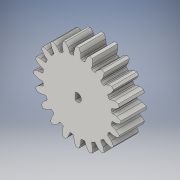
# Autodesk Inventor part: Pinion Gear
Saved by Autodesk Inventor 2016 (Build 200138000, 138)
## iProperties
Created: 2016-04-02
Part Number: Pinion Gear
Material: Generic
Document SubType Name: Modeling
Designer: amycroft3
Density: 1 g/cm^3
Appearance: White
Author: amycroft3
Autodesk Inventor part; units mm, degrees
ref_plane "YZ Plane" through (0, 0, 0) normal (1, 0, 0) x (0, 1, 0)
ref_plane "XZ Plane" through (0, 0, 0) normal (0, 1, 0) x (-1, 0, 0)
ref_plane "XY Plane" through (0, 0, 0) normal (0, 0, 1) x (1, 0, 0)
sketch "Sketch2" plane through (0, 0, 0) normal (0, 0, 1) x (1, 0, 0)
  spline S0 degree 3 poles (-17.8641, 1.7548) (-18.4191, 1.7613) (-18.9748, 1.7752) (-19.5187, 1.6705) (-19.6593, 1.6434) (-19.799, 1.6083) (-19.9383, 1.5692) knots 0 0 0 0 0.001655 0.001655 0.001655 0.002082 0.002082 0.002082 0.002082
  arc A0 (-19.9383, 1.5692) -> (-19.9383, -1.5692) centre (0, 0) ccw
  spline S1 degree 3 poles (-19.9383, -1.5692) (-19.7998, -1.6081) (-19.6596, -1.6433) (-19.5187, -1.6705) (-18.9722, -1.7757) (-18.418, -1.7613) (-17.8641, -1.7548) knots 0.002234 0.002234 0.002234 0.002234 0.002666 0.002666 0.002666 0.004341 0.004341 0.004341 0.004341
  arc A1 (-17.3622, -2.1921) -> (-17.8641, -1.7548) centre (-17.8582, -2.2548) ccw
  arc A2 (-17.3622, -2.1921) -> (-17.1898, -3.2804) centre (0, 0) ccw
  arc A3 (-17.532, -3.8514) -> (-17.1898, -3.2804) centre (-17.6809, -3.3741) ccw
  spline S2 degree 3 poles (-17.532, -3.8514) (-18.0619, -4.0167) (-18.5947, -4.1752) (-19.0796, -4.4429) (-19.2049, -4.5121) (-19.327, -4.5887) (-19.4474, -4.6689) knots 0 0 0 0 0.001655 0.001655 0.001655 0.002082 0.002082 0.002082 0.002082
  arc A4 (-19.4474, -4.6689) -> (-18.4776, -7.6537) centre (0, 0) ccw
  spline S3 degree 3 poles (-18.4776, -7.6537) (-18.3338, -7.6478) (-18.1895, -7.6381) (-18.0472, -7.6203) (-17.4949, -7.5515) (-16.9723, -7.3666) (-16.4475, -7.1892) knots 0.002234 0.002234 0.002234 0.002234 0.002666 0.002666 0.002666 0.004341 0.004341 0.004341 0.004341
  arc A5 (-15.835, -7.45) -> (-16.4475, -7.1892) centre (-16.2874, -7.6629) ccw
  arc A6 (-15.835, -7.45) -> (-15.3348, -8.4317) centre (0, 0) ccw
  arc A7 (-15.4838, -9.0806) -> (-15.3348, -8.4317) centre (-15.7729, -8.6727) ccw
  spline S4 degree 3 poles (-15.4838, -9.0806) (-15.9366, -9.4015) (-16.3944, -9.7169) (-16.7729, -10.1214) (-16.8707, -10.2259) (-16.9631, -10.3364) (-17.0528, -10.45) knots 0 0 0 0 0.001655 0.001655 0.001655 0.002082 0.002082 0.002082 0.002082
  arc A8 (-17.0528, -10.45) -> (-15.2081, -12.989) centre (0, 0) ccw
  spline S5 degree 3 poles (-15.2081, -12.989) (-15.0732, -12.939) (-14.939, -12.8851) (-14.8091, -12.8243) (-14.3051, -12.5882) (-13.8652, -12.2508) (-13.4209, -11.9199) knots 0.002234 0.002234 0.002234 0.002234 0.002666 0.002666 0.002666 0.004341 0.004341 0.004341 0.004341
  arc A9 (-12.7578, -11.9787) -> (-13.4209, -11.9199) centre (-13.1223, -12.3209) ccw
  arc A10 (-12.7578, -11.9787) -> (-11.9787, -12.7578) centre (0, 0) ccw
  arc A11 (-11.9199, -13.4209) -> (-11.9787, -12.7578) centre (-12.3209, -13.1223) ccw
  spline S6 degree 3 poles (-11.9199, -13.4209) (-12.2514, -13.8661) (-12.5893, -14.3075) (-12.8243, -14.8091) (-12.885, -14.9387) (-12.9387, -15.0724) (-12.989, -15.2081) knots 0 0 0 0 0.001655 0.001655 0.001655 0.002082 0.002082 0.002082 0.002082
  arc A12 (-12.989, -15.2081) -> (-10.45, -17.0528) centre (0, 0) ccw
  spline S7 degree 3 poles (-10.45, -17.0528) (-10.3371, -16.9636) (-10.2261, -16.8708) (-10.1214, -16.7729) (-9.715, -16.3926) (-9.4009, -15.9357) (-9.0806, -15.4838) knots 0.002234 0.002234 0.002234 0.002234 0.002666 0.002666 0.002666 0.004341 0.004341 0.004341 0.004341
  arc A13 (-8.4317, -15.3348) -> (-9.0806, -15.4838) centre (-8.6727, -15.7729) ccw
  arc A14 (-8.4317, -15.3348) -> (-7.45, -15.835) centre (0, 0) ccw
  arc A15 (-7.1892, -16.4475) -> (-7.45, -15.835) centre (-7.6629, -16.2874) ccw
  spline S8 degree 3 poles (-7.1892, -16.4475) (-7.3669, -16.9733) (-7.5519, -17.4975) (-7.6203, -18.0472) (-7.638, -18.1892) (-7.6478, -18.333) (-7.6537, -18.4776) knots 0 0 0 0 0.001655 0.001655 0.001655 0.002082 0.002082 0.002082 0.002082
  arc A16 (-7.6537, -18.4776) -> (-4.6689, -19.4474) centre (0, 0) ccw
  spline S9 degree 3 poles (-4.6689, -19.4474) (-4.5891, -19.3276) (-4.5122, -19.2052) (-4.4429, -19.0796) (-4.1739, -18.5923) (-4.0164, -18.0608) (-3.8514, -17.532) knots 0.002234 0.002234 0.002234 0.002234 0.002666 0.002666 0.002666 0.004341 0.004341 0.004341 0.004341
  arc A17 (-3.2804, -17.1898) -> (-3.8514, -17.532) centre (-3.3741, -17.6809) ccw
  arc A18 (-3.2804, -17.1898) -> (-2.1921, -17.3622) centre (0, 0) ccw
  arc A19 (-1.7548, -17.8641) -> (-2.1921, -17.3622) centre (-2.2548, -17.8582) ccw
  spline S10 degree 3 poles (-1.7548, -17.8641) (-1.7613, -18.4191) (-1.7752, -18.9748) (-1.6705, -19.5187) (-1.6434, -19.6593) (-1.6083, -19.799) (-1.5692, -19.9383) knots 0 0 0 0 0.001655 0.001655 0.001655 0.002082 0.002082 0.002082 0.002082
  arc A20 (-1.5692, -19.9383) -> (1.5692, -19.9383) centre (0, 0) ccw
  spline S11 degree 3 poles (1.5692, -19.9383) (1.6081, -19.7998) (1.6433, -19.6596) (1.6705, -19.5187) (1.7757, -18.9722) (1.7613, -18.418) (1.7548, -17.8641) knots 0.002234 0.002234 0.002234 0.002234 0.002666 0.002666 0.002666 0.004341 0.004341 0.004341 0.004341
  arc A21 (2.1921, -17.3622) -> (1.7548, -17.8641) centre (2.2548, -17.8582) ccw
  arc A22 (2.1921, -17.3622) -> (3.2804, -17.1898) centre (0, 0) ccw
  arc A23 (3.8514, -17.532) -> (3.2804, -17.1898) centre (3.3741, -17.6809) ccw
  spline S12 degree 3 poles (3.8514, -17.532) (4.0167, -18.0619) (4.1752, -18.5947) (4.4429, -19.0796) (4.5121, -19.2049) (4.5887, -19.327) (4.6689, -19.4474) knots 0 0 0 0 0.001655 0.001655 0.001655 0.002082 0.002082 0.002082 0.002082
  arc A24 (4.6689, -19.4474) -> (7.6537, -18.4776) centre (0, 0) ccw
  spline S13 degree 3 poles (7.6537, -18.4776) (7.6478, -18.3338) (7.6381, -18.1895) (7.6203, -18.0472) (7.5515, -17.4949) (7.3666, -16.9723) (7.1892, -16.4475) knots 0.002234 0.002234 0.002234 0.002234 0.002666 0.002666 0.002666 0.004341 0.004341 0.004341 0.004341
  arc A25 (7.45, -15.835) -> (7.1892, -16.4475) centre (7.6629, -16.2874) ccw
  arc A26 (7.45, -15.835) -> (8.4317, -15.3348) centre (0, 0) ccw
  arc A27 (9.0806, -15.4838) -> (8.4317, -15.3348) centre (8.6727, -15.7729) ccw
  spline S14 degree 3 poles (9.0806, -15.4838) (9.4015, -15.9366) (9.7169, -16.3944) (10.1214, -16.7729) (10.2259, -16.8707) (10.3364, -16.9631) (10.45, -17.0528) knots 0 0 0 0 0.001655 0.001655 0.001655 0.002082 0.002082 0.002082 0.002082
  arc A28 (10.45, -17.0528) -> (12.989, -15.2081) centre (0, 0) ccw
  spline S15 degree 3 poles (12.989, -15.2081) (12.939, -15.0732) (12.8851, -14.939) (12.8243, -14.8091) (12.5882, -14.3051) (12.2508, -13.8652) (11.9199, -13.4209) knots 0.002234 0.002234 0.002234 0.002234 0.002666 0.002666 0.002666 0.004341 0.004341 0.004341 0.004341
  arc A29 (11.9787, -12.7578) -> (11.9199, -13.4209) centre (12.3209, -13.1223) ccw
  arc A30 (11.9787, -12.7578) -> (12.7578, -11.9787) centre (0, 0) ccw
  arc A31 (13.4209, -11.9199) -> (12.7578, -11.9787) centre (13.1223, -12.3209) ccw
  spline S16 degree 3 poles (13.4209, -11.9199) (13.8661, -12.2514) (14.3075, -12.5893) (14.8091, -12.8243) (14.9387, -12.885) (15.0724, -12.9387) (15.2081, -12.989) knots 0 0 0 0 0.001655 0.001655 0.001655 0.002082 0.002082 0.002082 0.002082
  arc A32 (15.2081, -12.989) -> (17.0528, -10.45) centre (0, 0) ccw
  spline S17 degree 3 poles (17.0528, -10.45) (16.9636, -10.3371) (16.8708, -10.2261) (16.7729, -10.1214) (16.3926, -9.715) (15.9357, -9.4009) (15.4838, -9.0806) knots 0.002234 0.002234 0.002234 0.002234 0.002666 0.002666 0.002666 0.004341 0.004341 0.004341 0.004341
  arc A33 (15.3348, -8.4317) -> (15.4838, -9.0806) centre (15.7729, -8.6727) ccw
  arc A34 (15.3348, -8.4317) -> (15.835, -7.45) centre (0, 0) ccw
  arc A35 (16.4475, -7.1892) -> (15.835, -7.45) centre (16.2874, -7.6629) ccw
  spline S18 degree 3 poles (16.4475, -7.1892) (16.9733, -7.3669) (17.4975, -7.5519) (18.0472, -7.6203) (18.1892, -7.638) (18.333, -7.6478) (18.4776, -7.6537) knots 0 0 0 0 0.001655 0.001655 0.001655 0.002082 0.002082 0.002082 0.002082
  arc A36 (18.4776, -7.6537) -> (19.4474, -4.6689) centre (0, 0) ccw
  spline S19 degree 3 poles (19.4474, -4.6689) (19.3276, -4.5891) (19.2052, -4.5122) (19.0796, -4.4429) (18.5923, -4.1739) (18.0608, -4.0164) (17.532, -3.8514) knots 0.002234 0.002234 0.002234 0.002234 0.002666 0.002666 0.002666 0.004341 0.004341 0.004341 0.004341
  arc A37 (17.1898, -3.2804) -> (17.532, -3.8514) centre (17.6809, -3.3741) ccw
  arc A38 (17.1898, -3.2804) -> (17.3622, -2.1921) centre (0, 0) ccw
  arc A39 (17.8641, -1.7548) -> (17.3622, -2.1921) centre (17.8582, -2.2548) ccw
  spline S20 degree 3 poles (17.8641, -1.7548) (18.4191, -1.7613) (18.9748, -1.7752) (19.5187, -1.6705) (19.6593, -1.6434) (19.799, -1.6083) (19.9383, -1.5692) knots 0 0 0 0 0.001655 0.001655 0.001655 0.002082 0.002082 0.002082 0.002082
  arc A40 (19.9383, -1.5692) -> (19.9383, 1.5692) centre (0, 0) ccw
  spline S21 degree 3 poles (19.9383, 1.5692) (19.7998, 1.6081) (19.6596, 1.6433) (19.5187, 1.6705) (18.9722, 1.7757) (18.418, 1.7613) (17.8641, 1.7548) knots 0.002234 0.002234 0.002234 0.002234 0.002666 0.002666 0.002666 0.004341 0.004341 0.004341 0.004341
  arc A41 (17.3622, 2.1921) -> (17.8641, 1.7548) centre (17.8582, 2.2548) ccw
  arc A42 (17.3622, 2.1921) -> (17.1898, 3.2804) centre (0, 0) ccw
  arc A43 (17.532, 3.8514) -> (17.1898, 3.2804) centre (17.6809, 3.3741) ccw
  spline S22 degree 3 poles (17.532, 3.8514) (18.0619, 4.0167) (18.5947, 4.1752) (19.0796, 4.4429) (19.2049, 4.5121) (19.327, 4.5887) (19.4474, 4.6689) knots 0 0 0 0 0.001655 0.001655 0.001655 0.002082 0.002082 0.002082 0.002082
  arc A44 (19.4474, 4.6689) -> (18.4776, 7.6537) centre (0, 0) ccw
  spline S23 degree 3 poles (18.4776, 7.6537) (18.3338, 7.6478) (18.1895, 7.6381) (18.0472, 7.6203) (17.4949, 7.5515) (16.9723, 7.3666) (16.4475, 7.1892) knots 0.002234 0.002234 0.002234 0.002234 0.002666 0.002666 0.002666 0.004341 0.004341 0.004341 0.004341
  arc A45 (15.835, 7.45) -> (16.4475, 7.1892) centre (16.2874, 7.6629) ccw
  arc A46 (15.835, 7.45) -> (15.3348, 8.4317) centre (0, 0) ccw
  arc A47 (15.4838, 9.0806) -> (15.3348, 8.4317) centre (15.7729, 8.6727) ccw
  spline S24 degree 3 poles (15.4838, 9.0806) (15.9366, 9.4015) (16.3944, 9.7169) (16.7729, 10.1214) (16.8707, 10.2259) (16.9631, 10.3364) (17.0528, 10.45) knots 0 0 0 0 0.001655 0.001655 0.001655 0.002082 0.002082 0.002082 0.002082
  arc A48 (17.0528, 10.45) -> (15.2081, 12.989) centre (0, 0) ccw
  spline S25 degree 3 poles (15.2081, 12.989) (15.0732, 12.939) (14.939, 12.8851) (14.8091, 12.8243) (14.3051, 12.5882) (13.8652, 12.2508) (13.4209, 11.9199) knots 0.002234 0.002234 0.002234 0.002234 0.002666 0.002666 0.002666 0.004341 0.004341 0.004341 0.004341
  arc A49 (12.7578, 11.9787) -> (13.4209, 11.9199) centre (13.1223, 12.3209) ccw
  arc A50 (12.7578, 11.9787) -> (11.9787, 12.7578) centre (0, 0) ccw
  arc A51 (11.9199, 13.4209) -> (11.9787, 12.7578) centre (12.3209, 13.1223) ccw
  spline S26 degree 3 poles (11.9199, 13.4209) (12.2514, 13.8661) (12.5893, 14.3075) (12.8243, 14.8091) (12.885, 14.9387) (12.9387, 15.0724) (12.989, 15.2081) knots 0 0 0 0 0.001655 0.001655 0.001655 0.002082 0.002082 0.002082 0.002082
  arc A52 (12.989, 15.2081) -> (10.45, 17.0528) centre (0, 0) ccw
  spline S27 degree 3 poles (10.45, 17.0528) (10.3371, 16.9636) (10.2261, 16.8708) (10.1214, 16.7729) (9.715, 16.3926) (9.4009, 15.9357) (9.0806, 15.4838) knots 0.002234 0.002234 0.002234 0.002234 0.002666 0.002666 0.002666 0.004341 0.004341 0.004341 0.004341
  arc A53 (8.4317, 15.3348) -> (9.0806, 15.4838) centre (8.6727, 15.7729) ccw
  arc A54 (8.4317, 15.3348) -> (7.45, 15.835) centre (0, 0) ccw
  arc A55 (7.1892, 16.4475) -> (7.45, 15.835) centre (7.6629, 16.2874) ccw
  spline S28 degree 3 poles (7.1892, 16.4475) (7.3669, 16.9733) (7.5519, 17.4975) (7.6203, 18.0472) (7.638, 18.1892) (7.6478, 18.333) (7.6537, 18.4776) knots 0 0 0 0 0.001655 0.001655 0.001655 0.002082 0.002082 0.002082 0.002082
  arc A56 (7.6537, 18.4776) -> (4.6689, 19.4474) centre (0, 0) ccw
  spline S29 degree 3 poles (4.6689, 19.4474) (4.5891, 19.3276) (4.5122, 19.2052) (4.4429, 19.0796) (4.1739, 18.5923) (4.0164, 18.0608) (3.8514, 17.532) knots 0.002234 0.002234 0.002234 0.002234 0.002666 0.002666 0.002666 0.004341 0.004341 0.004341 0.004341
  arc A57 (3.2804, 17.1898) -> (3.8514, 17.532) centre (3.3741, 17.6809) ccw
  arc A58 (3.2804, 17.1898) -> (2.1921, 17.3622) centre (0, 0) ccw
  arc A59 (1.7548, 17.8641) -> (2.1921, 17.3622) centre (2.2548, 17.8582) ccw
  spline S30 degree 3 poles (1.7548, 17.8641) (1.7613, 18.4191) (1.7752, 18.9748) (1.6705, 19.5187) (1.6434, 19.6593) (1.6083, 19.799) (1.5692, 19.9383) knots 0 0 0 0 0.001655 0.001655 0.001655 0.002082 0.002082 0.002082 0.002082
  arc A60 (1.5692, 19.9383) -> (-1.5692, 19.9383) centre (0, 0) ccw
  spline S31 degree 3 poles (-1.5692, 19.9383) (-1.6081, 19.7998) (-1.6433, 19.6596) (-1.6705, 19.5187) (-1.7757, 18.9722) (-1.7613, 18.418) (-1.7548, 17.8641) knots 0.002234 0.002234 0.002234 0.002234 0.002666 0.002666 0.002666 0.004341 0.004341 0.004341 0.004341
  arc A61 (-2.1921, 17.3622) -> (-1.7548, 17.8641) centre (-2.2548, 17.8582) ccw
  arc A62 (-2.1921, 17.3622) -> (-3.2804, 17.1898) centre (0, 0) ccw
  arc A63 (-3.8514, 17.532) -> (-3.2804, 17.1898) centre (-3.3741, 17.6809) ccw
  spline S32 degree 3 poles (-3.8514, 17.532) (-4.0167, 18.0619) (-4.1752, 18.5947) (-4.4429, 19.0796) (-4.5121, 19.2049) (-4.5887, 19.327) (-4.6689, 19.4474) knots 0 0 0 0 0.001655 0.001655 0.001655 0.002082 0.002082 0.002082 0.002082
  arc A64 (-4.6689, 19.4474) -> (-7.6537, 18.4776) centre (0, 0) ccw
  spline S33 degree 3 poles (-7.6537, 18.4776) (-7.6478, 18.3338) (-7.6381, 18.1895) (-7.6203, 18.0472) (-7.5515, 17.4949) (-7.3666, 16.9723) (-7.1892, 16.4475) knots 0.002234 0.002234 0.002234 0.002234 0.002666 0.002666 0.002666 0.004341 0.004341 0.004341 0.004341
  arc A65 (-7.45, 15.835) -> (-7.1892, 16.4475) centre (-7.6629, 16.2874) ccw
  arc A66 (-7.45, 15.835) -> (-8.4317, 15.3348) centre (0, 0) ccw
  arc A67 (-9.0806, 15.4838) -> (-8.4317, 15.3348) centre (-8.6727, 15.7729) ccw
  spline S34 degree 3 poles (-9.0806, 15.4838) (-9.4015, 15.9366) (-9.7169, 16.3944) (-10.1214, 16.7729) (-10.2259, 16.8707) (-10.3364, 16.9631) (-10.45, 17.0528) knots 0 0 0 0 0.001655 0.001655 0.001655 0.002082 0.002082 0.002082 0.002082
  arc A68 (-10.45, 17.0528) -> (-12.989, 15.2081) centre (0, 0) ccw
  spline S35 degree 3 poles (-12.989, 15.2081) (-12.939, 15.0732) (-12.8851, 14.939) (-12.8243, 14.8091) (-12.5882, 14.3051) (-12.2508, 13.8652) (-11.9199, 13.4209) knots 0.002234 0.002234 0.002234 0.002234 0.002666 0.002666 0.002666 0.004341 0.004341 0.004341 0.004341
  arc A69 (-11.9787, 12.7578) -> (-11.9199, 13.4209) centre (-12.3209, 13.1223) ccw
  arc A70 (-11.9787, 12.7578) -> (-12.7578, 11.9787) centre (0, 0) ccw
  arc A71 (-13.4209, 11.9199) -> (-12.7578, 11.9787) centre (-13.1223, 12.3209) ccw
  spline S36 degree 3 poles (-13.4209, 11.9199) (-13.8661, 12.2514) (-14.3075, 12.5893) (-14.8091, 12.8243) (-14.9387, 12.885) (-15.0724, 12.9387) (-15.2081, 12.989) knots 0 0 0 0 0.001655 0.001655 0.001655 0.002082 0.002082 0.002082 0.002082
  arc A72 (-15.2081, 12.989) -> (-17.0528, 10.45) centre (0, 0) ccw
  spline S37 degree 3 poles (-17.0528, 10.45) (-16.9636, 10.3371) (-16.8708, 10.2261) (-16.7729, 10.1214) (-16.3926, 9.715) (-15.9357, 9.4009) (-15.4838, 9.0806) knots 0.002234 0.002234 0.002234 0.002234 0.002666 0.002666 0.002666 0.004341 0.004341 0.004341 0.004341
  arc A73 (-15.3348, 8.4317) -> (-15.4838, 9.0806) centre (-15.7729, 8.6727) ccw
  arc A74 (-15.3348, 8.4317) -> (-15.835, 7.45) centre (0, 0) ccw
  arc A75 (-16.4475, 7.1892) -> (-15.835, 7.45) centre (-16.2874, 7.6629) ccw
  spline S38 degree 3 poles (-16.4475, 7.1892) (-16.9733, 7.3669) (-17.4975, 7.5519) (-18.0472, 7.6203) (-18.1892, 7.638) (-18.333, 7.6478) (-18.4776, 7.6537) knots 0 0 0 0 0.001655 0.001655 0.001655 0.002082 0.002082 0.002082 0.002082
  arc A76 (-18.4776, 7.6537) -> (-19.4474, 4.6689) centre (0, 0) ccw
  spline S39 degree 3 poles (-19.4474, 4.6689) (-19.3276, 4.5891) (-19.2052, 4.5122) (-19.0796, 4.4429) (-18.5923, 4.1739) (-18.0608, 4.0164) (-17.532, 3.8514) knots 0.002234 0.002234 0.002234 0.002234 0.002666 0.002666 0.002666 0.004341 0.004341 0.004341 0.004341
  arc A77 (-17.1898, 3.2804) -> (-17.532, 3.8514) centre (-17.6809, 3.3741) ccw
  arc A78 (-17.1898, 3.2804) -> (-17.3622, 2.1921) centre (0, 0) ccw
  arc A79 (-17.8641, 1.7548) -> (-17.3622, 2.1921) centre (-17.8582, 2.2548) ccw
  arc A80 (-15.2081, 12.989) -> (-17.0528, 10.45) centre (0, 0) ccw
  spline S40 degree 3 poles (-17.3812, 13.4869) (-17.0145, 13.4452) (-16.6476, 13.3855) (-15.9177, 13.2226) (-15.5627, 13.1203) (-15.2081, 12.989) knots -0.225972 -0.225972 -0.225972 -0.225972 -0.113443 -0.113443 -0.000001 -0.000001 -0.000001 -0.000001
  arc A81 (-17.3812, 13.4869) -> (-18.1978, 12.3628) centre (0, 0) ccw
  spline S41 degree 3 poles (-17.0528, 10.45) (-17.2873, 10.7466) (-17.4943, 11.0526) (-17.8748, 11.6964) (-18.045, 12.027) (-18.1978, 12.3628) knots -0.22563 -0.22563 -0.22563 -0.22563 -0.112359 -0.112359 0 0 0 0
  arc A82 (-18.4776, 7.6537) -> (-19.4474, 4.6689) centre (0, 0) ccw
  spline S42 degree 3 poles (-20.6981, 7.4557) (-20.3366, 7.5294) (-19.9691, 7.586) (-19.2247, 7.6566) (-18.8554, 7.669) (-18.4776, 7.6537) knots -0.225972 -0.225972 -0.225972 -0.225972 -0.113443 -0.113443 -0.000001 -0.000001 -0.000001 -0.000001
  arc A83 (-20.6981, 7.4557) -> (-21.1275, 6.1343) centre (0, 0) ccw
  spline S43 degree 3 poles (-19.4474, 4.6689) (-19.7621, 4.8786) (-20.0535, 5.1057) (-20.6143, 5.6003) (-20.8783, 5.8621) (-21.1275, 6.1343) knots -0.22563 -0.22563 -0.22563 -0.22563 -0.112359 -0.112359 0 0 0 0
  arc A84 (-19.9383, 1.5692) -> (-19.9383, -1.5692) centre (0, 0) ccw
  spline S44 degree 3 poles (-21.989, 0.6947) (-21.668, 0.8765) (-21.336, 1.0439) (-20.6498, 1.3411) (-20.3024, 1.467) (-19.9383, 1.5692) knots -0.225972 -0.225972 -0.225972 -0.225972 -0.113443 -0.113443 -0.000001 -0.000001 -0.000001 -0.000001
  arc A85 (-21.989, 0.6947) -> (-21.989, -0.6947) centre (0, 0) ccw
  spline S45 degree 3 poles (-19.9383, -1.5692) (-20.3024, -1.467) (-20.6498, -1.3411) (-21.336, -1.0439) (-21.668, -0.8765) (-21.989, -0.6947) knots -0.22563 -0.22563 -0.22563 -0.22563 -0.112359 -0.112359 0 0 0 0
  arc A86 (-19.4474, -4.6689) -> (-18.4776, -7.6537) centre (0, 0) ccw
  arc A87 (-19.4474, -4.6689) -> (-18.4776, -7.6537) centre (0, 0) ccw
  spline S46 degree 3 poles (-21.1275, -6.1343) (-20.8783, -5.8621) (-20.6143, -5.6003) (-20.0535, -5.1057) (-19.7621, -4.8786) (-19.4474, -4.6689) knots -0.225972 -0.225972 -0.225972 -0.225972 -0.113443 -0.113443 -0.000001 -0.000001 -0.000001 -0.000001
  arc A88 (-21.1275, -6.1343) -> (-20.6981, -7.4557) centre (0, 0) ccw
  spline S47 degree 3 poles (-18.4776, -7.6537) (-18.8554, -7.669) (-19.2247, -7.6566) (-19.9691, -7.586) (-20.3366, -7.5294) (-20.6981, -7.4557) knots -0.22563 -0.22563 -0.22563 -0.22563 -0.112359 -0.112359 0 0 0 0
  arc A89 (-17.0528, -10.45) -> (-15.2081, -12.989) centre (0, 0) ccw
  spline S48 degree 3 poles (-18.1978, -12.3628) (-18.045, -12.027) (-17.8748, -11.6964) (-17.4943, -11.0526) (-17.2873, -10.7466) (-17.0528, -10.45) knots -0.225972 -0.225972 -0.225972 -0.225972 -0.113443 -0.113443 -0.000001 -0.000001 -0.000001 -0.000001
  arc A90 (-18.1978, -12.3628) -> (-17.3812, -13.4869) centre (0, 0) ccw
  spline S49 degree 3 poles (-15.2081, -12.989) (-15.5627, -13.1203) (-15.9177, -13.2226) (-16.6476, -13.3855) (-17.0145, -13.4452) (-17.3812, -13.4869) knots -0.22563 -0.22563 -0.22563 -0.22563 -0.112359 -0.112359 0 0 0 0
  arc A91 (-12.989, -15.2081) -> (-10.45, -17.0528) centre (0, 0) ccw
  spline S50 degree 3 poles (-13.4869, -17.3812) (-13.4452, -17.0145) (-13.3855, -16.6476) (-13.2226, -15.9177) (-13.1203, -15.5627) (-12.989, -15.2081) knots -0.225972 -0.225972 -0.225972 -0.225972 -0.113443 -0.113443 -0.000001 -0.000001 -0.000001 -0.000001
  arc A92 (-13.4869, -17.3812) -> (-12.3628, -18.1978) centre (0, 0) ccw
  spline S51 degree 3 poles (-10.45, -17.0528) (-10.7466, -17.2873) (-11.0526, -17.4943) (-11.6964, -17.8748) (-12.027, -18.045) (-12.3628, -18.1978) knots -0.22563 -0.22563 -0.22563 -0.22563 -0.112359 -0.112359 0 0 0 0
  arc A93 (-7.6537, -18.4776) -> (-4.6689, -19.4474) centre (0, 0) ccw
  spline S52 degree 3 poles (-7.4557, -20.6981) (-7.5294, -20.3366) (-7.586, -19.9691) (-7.6566, -19.2247) (-7.669, -18.8554) (-7.6537, -18.4776) knots -0.225972 -0.225972 -0.225972 -0.225972 -0.113443 -0.113443 -0.000001 -0.000001 -0.000001 -0.000001
  arc A94 (-7.4557, -20.6981) -> (-6.1343, -21.1275) centre (0, 0) ccw
  spline S53 degree 3 poles (-4.6689, -19.4474) (-4.8786, -19.7621) (-5.1057, -20.0535) (-5.6003, -20.6143) (-5.8621, -20.8783) (-6.1343, -21.1275) knots -0.22563 -0.22563 -0.22563 -0.22563 -0.112359 -0.112359 0 0 0 0
  arc A95 (-1.5692, -19.9383) -> (1.5692, -19.9383) centre (0, 0) ccw
  spline S54 degree 3 poles (-0.6947, -21.989) (-0.8765, -21.668) (-1.0439, -21.336) (-1.3411, -20.6498) (-1.467, -20.3024) (-1.5692, -19.9383) knots -0.225972 -0.225972 -0.225972 -0.225972 -0.113443 -0.113443 -0.000001 -0.000001 -0.000001 -0.000001
  arc A96 (-0.6947, -21.989) -> (0.6947, -21.989) centre (0, 0) ccw
  spline S55 degree 3 poles (1.5692, -19.9383) (1.467, -20.3024) (1.3411, -20.6498) (1.0439, -21.336) (0.8765, -21.668) (0.6947, -21.989) knots -0.22563 -0.22563 -0.22563 -0.22563 -0.112359 -0.112359 0 0 0 0
  arc A97 (4.6689, -19.4474) -> (7.6537, -18.4776) centre (0, 0) ccw
  spline S56 degree 3 poles (6.1343, -21.1275) (5.8621, -20.8783) (5.6003, -20.6143) (5.1057, -20.0535) (4.8786, -19.7621) (4.6689, -19.4474) knots -0.225972 -0.225972 -0.225972 -0.225972 -0.113443 -0.113443 -0.000001 -0.000001 -0.000001 -0.000001
  arc A98 (6.1343, -21.1275) -> (7.4557, -20.6981) centre (0, 0) ccw
  spline S57 degree 3 poles (7.6537, -18.4776) (7.669, -18.8554) (7.6566, -19.2247) (7.586, -19.9691) (7.5294, -20.3366) (7.4557, -20.6981) knots -0.22563 -0.22563 -0.22563 -0.22563 -0.112359 -0.112359 0 0 0 0
  arc A99 (10.45, -17.0528) -> (12.989, -15.2081) centre (0, 0) ccw
  spline S58 degree 3 poles (12.3628, -18.1978) (12.027, -18.045) (11.6964, -17.8748) (11.0526, -17.4943) (10.7466, -17.2873) (10.45, -17.0528) knots -0.225972 -0.225972 -0.225972 -0.225972 -0.113443 -0.113443 -0.000001 -0.000001 -0.000001 -0.000001
  arc A100 (12.3628, -18.1978) -> (13.4869, -17.3812) centre (0, 0) ccw
  spline S59 degree 3 poles (12.989, -15.2081) (13.1203, -15.5627) (13.2226, -15.9177) (13.3855, -16.6476) (13.4452, -17.0145) (13.4869, -17.3812) knots -0.22563 -0.22563 -0.22563 -0.22563 -0.112359 -0.112359 0 0 0 0
  arc A101 (15.2081, -12.989) -> (17.0528, -10.45) centre (0, 0) ccw
  spline S60 degree 3 poles (17.3812, -13.4869) (17.0145, -13.4452) (16.6476, -13.3855) (15.9177, -13.2226) (15.5627, -13.1203) (15.2081, -12.989) knots -0.225972 -0.225972 -0.225972 -0.225972 -0.113443 -0.113443 -0.000001 -0.000001 -0.000001 -0.000001
  arc A102 (17.3812, -13.4869) -> (18.1978, -12.3628) centre (0, 0) ccw
  spline S61 degree 3 poles (17.0528, -10.45) (17.2873, -10.7466) (17.4943, -11.0526) (17.8748, -11.6964) (18.045, -12.027) (18.1978, -12.3628) knots -0.22563 -0.22563 -0.22563 -0.22563 -0.112359 -0.112359 0 0 0 0
  arc A103 (18.4776, -7.6537) -> (19.4474, -4.6689) centre (0, 0) ccw
  spline S62 degree 3 poles (20.6981, -7.4557) (20.3366, -7.5294) (19.9691, -7.586) (19.2247, -7.6566) (18.8554, -7.669) (18.4776, -7.6537) knots -0.225972 -0.225972 -0.225972 -0.225972 -0.113443 -0.113443 -0.000001 -0.000001 -0.000001 -0.000001
  arc A104 (20.6981, -7.4557) -> (21.1275, -6.1343) centre (0, 0) ccw
  spline S63 degree 3 poles (19.4474, -4.6689) (19.7621, -4.8786) (20.0535, -5.1057) (20.6143, -5.6003) (20.8783, -5.8621) (21.1275, -6.1343) knots -0.22563 -0.22563 -0.22563 -0.22563 -0.112359 -0.112359 0 0 0 0
  arc A105 (19.9383, -1.5692) -> (19.9383, 1.5692) centre (0, 0) ccw
  spline S64 degree 3 poles (21.989, -0.6947) (21.668, -0.8765) (21.336, -1.0439) (20.6498, -1.3411) (20.3024, -1.467) (19.9383, -1.5692) knots -0.225972 -0.225972 -0.225972 -0.225972 -0.113443 -0.113443 -0.000001 -0.000001 -0.000001 -0.000001
  arc A106 (21.989, -0.6947) -> (21.989, 0.6947) centre (0, 0) ccw
  spline S65 degree 3 poles (19.9383, 1.5692) (20.3024, 1.467) (20.6498, 1.3411) (21.336, 1.0439) (21.668, 0.8765) (21.989, 0.6947) knots -0.22563 -0.22563 -0.22563 -0.22563 -0.112359 -0.112359 0 0 0 0
  arc A107 (19.4474, 4.6689) -> (18.4776, 7.6537) centre (0, 0) ccw
  spline S66 degree 3 poles (21.1275, 6.1343) (20.8783, 5.8621) (20.6143, 5.6003) (20.0535, 5.1057) (19.7621, 4.8786) (19.4474, 4.6689) knots -0.225972 -0.225972 -0.225972 -0.225972 -0.113443 -0.113443 -0.000001 -0.000001 -0.000001 -0.000001
  arc A108 (21.1275, 6.1343) -> (20.6981, 7.4557) centre (0, 0) ccw
  spline S67 degree 3 poles (18.4776, 7.6537) (18.8554, 7.669) (19.2247, 7.6566) (19.9691, 7.586) (20.3366, 7.5294) (20.6981, 7.4557) knots -0.22563 -0.22563 -0.22563 -0.22563 -0.112359 -0.112359 0 0 0 0
  arc A109 (17.0528, 10.45) -> (15.2081, 12.989) centre (0, 0) ccw
  spline S68 degree 3 poles (18.1978, 12.3628) (18.045, 12.027) (17.8748, 11.6964) (17.4943, 11.0526) (17.2873, 10.7466) (17.0528, 10.45) knots -0.225972 -0.225972 -0.225972 -0.225972 -0.113443 -0.113443 -0.000001 -0.000001 -0.000001 -0.000001
  arc A110 (18.1978, 12.3628) -> (17.3812, 13.4869) centre (0, 0) ccw
  spline S69 degree 3 poles (15.2081, 12.989) (15.5627, 13.1203) (15.9177, 13.2226) (16.6476, 13.3855) (17.0145, 13.4452) (17.3812, 13.4869) knots -0.22563 -0.22563 -0.22563 -0.22563 -0.112359 -0.112359 0 0 0 0
  spline S70 degree 3 poles (10.45, 17.0528) (10.7466, 17.2873) (11.0526, 17.4943) (11.6964, 17.8748) (12.027, 18.045) (12.3628, 18.1978) knots -0.22563 -0.22563 -0.22563 -0.22563 -0.112359 -0.112359 0 0 0 0
  arc A111 (12.989, 15.2081) -> (10.45, 17.0528) centre (0, 0) ccw
  spline S71 degree 3 poles (13.4869, 17.3812) (13.4452, 17.0145) (13.3855, 16.6476) (13.2226, 15.9177) (13.1203, 15.5627) (12.989, 15.2081) knots -0.225972 -0.225972 -0.225972 -0.225972 -0.113443 -0.113443 -0.000001 -0.000001 -0.000001 -0.000001
  arc A112 (13.4869, 17.3812) -> (12.3628, 18.1978) centre (0, 0) ccw
  spline S72 degree 3 poles (10.45, 17.0528) (10.7466, 17.2873) (11.0526, 17.4943) (11.6964, 17.8748) (12.027, 18.045) (12.3628, 18.1978) knots -0.22563 -0.22563 -0.22563 -0.22563 -0.112359 -0.112359 0 0 0 0
  arc A113 (7.6537, 18.4776) -> (4.6689, 19.4474) centre (0, 0) ccw
  spline S73 degree 3 poles (7.4557, 20.6981) (7.5294, 20.3366) (7.586, 19.9691) (7.6566, 19.2247) (7.669, 18.8554) (7.6537, 18.4776) knots -0.225972 -0.225972 -0.225972 -0.225972 -0.113443 -0.113443 -0.000001 -0.000001 -0.000001 -0.000001
  arc A114 (7.4557, 20.6981) -> (6.1343, 21.1275) centre (0, 0) ccw
  spline S74 degree 3 poles (4.6689, 19.4474) (4.8786, 19.7621) (5.1057, 20.0535) (5.6003, 20.6143) (5.8621, 20.8783) (6.1343, 21.1275) knots -0.22563 -0.22563 -0.22563 -0.22563 -0.112359 -0.112359 0 0 0 0
  arc A115 (1.5692, 19.9383) -> (-1.5692, 19.9383) centre (0, 0) ccw
  spline S75 degree 3 poles (0.6947, 21.989) (0.8765, 21.668) (1.0439, 21.336) (1.3411, 20.6498) (1.467, 20.3024) (1.5692, 19.9383) knots -0.225972 -0.225972 -0.225972 -0.225972 -0.113443 -0.113443 -0.000001 -0.000001 -0.000001 -0.000001
  arc A116 (0.6947, 21.989) -> (-0.6947, 21.989) centre (0, 0) ccw
  spline S76 degree 3 poles (-1.5692, 19.9383) (-1.467, 20.3024) (-1.3411, 20.6498) (-1.0439, 21.336) (-0.8765, 21.668) (-0.6947, 21.989) knots -0.22563 -0.22563 -0.22563 -0.22563 -0.112359 -0.112359 0 0 0 0
  arc A117 (-4.6689, 19.4474) -> (-7.6537, 18.4776) centre (0, 0) ccw
  spline S77 degree 3 poles (-6.1343, 21.1275) (-5.8621, 20.8783) (-5.6003, 20.6143) (-5.1057, 20.0535) (-4.8786, 19.7621) (-4.6689, 19.4474) knots -0.225972 -0.225972 -0.225972 -0.225972 -0.113443 -0.113443 -0.000001 -0.000001 -0.000001 -0.000001
  arc A118 (-6.1343, 21.1275) -> (-7.4557, 20.6981) centre (0, 0) ccw
  spline S78 degree 3 poles (-7.6537, 18.4776) (-7.669, 18.8554) (-7.6566, 19.2247) (-7.586, 19.9691) (-7.5294, 20.3366) (-7.4557, 20.6981) knots -0.22563 -0.22563 -0.22563 -0.22563 -0.112359 -0.112359 0 0 0 0
  arc A119 (-10.45, 17.0528) -> (-12.989, 15.2081) centre (0, 0) ccw
  spline S79 degree 3 poles (-12.3628, 18.1978) (-12.027, 18.045) (-11.6964, 17.8748) (-11.0526, 17.4943) (-10.7466, 17.2873) (-10.45, 17.0528) knots -0.225972 -0.225972 -0.225972 -0.225972 -0.113443 -0.113443 -0.000001 -0.000001 -0.000001 -0.000001
  arc A120 (-12.3628, 18.1978) -> (-13.4869, 17.3812) centre (0, 0) ccw
  spline S80 degree 3 poles (-12.989, 15.2081) (-13.1203, 15.5627) (-13.2226, 15.9177) (-13.3855, 16.6476) (-13.4452, 17.0145) (-13.4869, 17.3812) knots -0.22563 -0.22563 -0.22563 -0.22563 -0.112359 -0.112359 0 0 0 0
  constraints: 242 point on circle, 121 centre point, 243 other
extrude "Extrusion1" add sketch "Sketch2" along normal blind 12.7
sketch "Sketch3" plane through (0, 0, 12.7) normal (0, 0, 1) x (1, 0, 0)
  arc A0 (-1.016, -1.7227) -> (-1.016, 1.7227) centre (0, 0) ccw
  line L0 (-1.016, 1.7227) -> (-1.016, -1.7227)
  dimension "d2" = 4
  dimension "d3" = 1.016
  constraints: 2 end point, 2 point on circle, 1 centre point, 1 coincident, 1 vertical
  measures "d2" diameter of A0
  measures "d3" distance from line of L0 point (0, 0)
extrude "Extrusion2" cut sketch "Sketch3" against normal blind 9.398
sketch "Sketch4" plane through (0, 0, 12.7) normal (0, 0, 1) x (1, 0, 0)
  arc A0 (12.3628, -18.1978) -> (13.4869, -17.3812) centre (0, 0) ccw projected
  circle A1 centre (0, 0) radius 22
  constraints: 1 coincident, 3 other
sketch "Sketch5" plane through (0, 0, 0) normal (0, 0, -1) x (-1, 0, 0)
  arc A0 (17.3812, -13.4869) -> (18.1978, -12.3628) centre (0, 0) ccw projected
  circle A1 centre (0, 0) radius 22
  constraints: 1 coincident, 3 other
body "Solid1"
